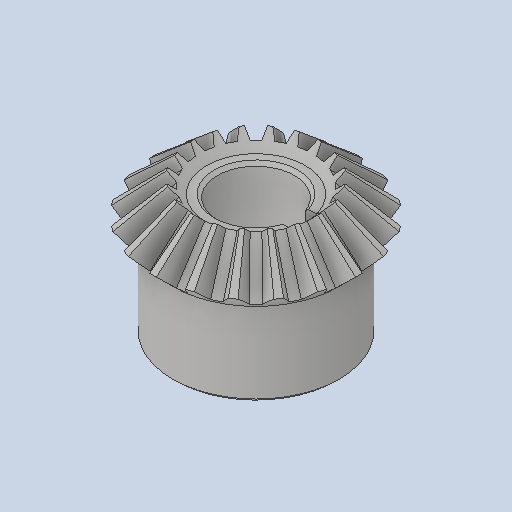
# Autodesk Inventor part: SMB1_5-201p_On
Saved by Autodesk Inventor 2025.2 (Build 292293000, 293)
## iProperties
Category: PARTsolutions
Company: KHK
Created: 2023-02-24
Part Number: SMB1_5-201p_On
Material: Generic
Catalog Web Link: www.cadenas.de
Description: SMB-
Vendor: KHK
Document SubType Name: Modeling
Designer: psAdmin
Manufacturer: KHK
Mass: 7.93706 g
Surface Area: 38.4961 cm^2
Volume: 7.93706 cm^3
Density: 1 g/cm^3
Appearance: PSOLRGB-175-175-175
PSOL_IDENT_0: {$CADENAS_DATA/23d-libs/khk/miter_gears/smb.prj},178 {VTYP=3D},{NB=SMB1.5-201p_On},{LINA=SMB1.5-20},
PSOL_IDENT_1: {NN=SMB},{DATE=06.10.2022 23:14:45},{GEOMDATE=24.04.2019 13:37:34},{VERSION=},{LINEID=300},{WBVAR=CO
PSOL_IDENT_2: MBINATION,TOOTH},{WBNUMERIC=}  {NB=SMB1.5-201p_On},{LINA=SMB1.5-20},{KT=DUMMY},{CN=SMB1.5-20},{COMBI
PSOL_IDENT_3: NATION=1},{VERS=2},{M=1.5},{Z=20},{A=12},{B=26},{C=30},{D=32.12},{E=30},{F=21.24},{G=16.06},{H=13.0}
PSOL_IDENT_4: ,{I=19},{J=8},{K=15.37},{L=49.80},{KYW=4x1.8},{KW=4},{KD=1.8},{TDM=6.50},{TS=M5},{S=B3},{PN=SMB1.5-2
PSOL_IDENT_5: 0},{WMF=B3004.WMF},{X=0.5},{Y=0.5},{TSNDM=5},{TOOTH=On}
NB: SMB1.5-201p_On
NN: SMB
NBSYN: $CN.$COMBINATION.p_$TOOTH.
LINA: SMB1.5-20
CATALOG: KHK
CN: SMB1.5-20
COMBINATION: Single
VERS: 2
M: 1.5
Z: 20
A: 12
B: 26
C: 30
D: 32.12
E: 30
F: 21.24
G: 16.06
H: 13
I: 19
J: 8
K: 15.37
L: 49.8
KYW: 4x1.8
KW: 4
KD: 1.8
TDM: 6.5
TS: M5
S: B3
PN: SMB1.5-20
WMF: B3004.WMF
X: 0.5
Y: 0.5
TSNDM: 5
TOOTH: On
SUPPLIER: KHK
ARTICLENO: SMB1.5-201p_On
BOMINFO: SMB1.5-20
CREATOR: CADENAS GmbH
Title: SMB1.5-20
Author: Cadenas PARTsolutions
Autodesk Inventor part; units mm, degrees
sketch "Sketch_6" plane through (0, -17, 0) normal (0, 1, 0) x (1, 0, 0)
  arc A0 (-0.5083, 20.2214) -> (-1.5864, 14.3695) centre (19.5954, 13.4924) ccw
  arc A1 (-1.5864, 14.3695) -> (-2.9317, 14.1564) centre (0, 0) ccw
  arc A2 (-2.9317, 14.1564) -> (-5.7653, 19.3888) centre (-22.8058, 6.7768) ccw
  arc A3 (-5.7653, 19.3888) -> (-6.7322, 19.0746) centre (0, 0) ccw
  arc A4 (-6.7322, 19.0746) -> (-5.9492, 13.176) centre (14.467, 18.8874) ccw
  arc A5 (-5.9492, 13.176) -> (-7.1627, 12.5576) centre (0, 0) ccw
  arc A6 (-7.1627, 12.5576) -> (-11.4746, 16.6582) centre (-23.7837, -0.6023) ccw
  arc A7 (-11.4746, 16.6582) -> (-12.2971, 16.0607) centre (0, 0) ccw
  arc A8 (-12.2971, 16.0607) -> (-9.7296, 10.6927) centre (7.9224, 22.4335) ccw
  arc A9 (-9.7296, 10.6927) -> (-10.6927, 9.7296) centre (0, 0) ccw
  arc A10 (-10.6927, 9.7296) -> (-16.0607, 12.2971) centre (-22.4335, -7.9224) ccw
  arc A11 (-16.0607, 12.2971) -> (-16.6582, 11.4746) centre (0, 0) ccw
  arc A12 (-16.6582, 11.4746) -> (-12.5576, 7.1627) centre (0.6023, 23.7837) ccw
  arc A13 (-12.5576, 7.1627) -> (-13.176, 5.9492) centre (0, 0) ccw
  arc A14 (-13.176, 5.9492) -> (-19.0746, 6.7322) centre (-18.8874, -14.467) ccw
  arc A15 (-19.0746, 6.7322) -> (-19.3888, 5.7653) centre (0, 0) ccw
  arc A16 (-19.3888, 5.7653) -> (-14.1564, 2.9317) centre (-6.7768, 22.8058) ccw
  arc A17 (-14.1564, 2.9317) -> (-14.3695, 1.5864) centre (0, 0) ccw
  arc A18 (-14.3695, 1.5864) -> (-20.2214, 0.5083) centre (-13.4924, -19.5954) ccw
  arc A19 (-20.2214, 0.5083) -> (-20.2214, -0.5083) centre (0, 0) ccw
  arc A20 (-20.2214, -0.5083) -> (-14.3695, -1.5864) centre (-13.4924, 19.5954) ccw
  arc A21 (-14.3695, -1.5864) -> (-14.1564, -2.9317) centre (0, 0) ccw
  arc A22 (-14.1564, -2.9317) -> (-19.3888, -5.7653) centre (-6.7768, -22.8058) ccw
  arc A23 (-19.3888, -5.7653) -> (-19.0746, -6.7322) centre (0, 0) ccw
  arc A24 (-19.0746, -6.7322) -> (-13.176, -5.9492) centre (-18.8874, 14.467) ccw
  arc A25 (-13.176, -5.9492) -> (-12.5576, -7.1627) centre (0, 0) ccw
  arc A26 (-12.5576, -7.1627) -> (-16.6582, -11.4746) centre (0.6023, -23.7837) ccw
  arc A27 (-16.6582, -11.4746) -> (-16.0607, -12.2971) centre (0, 0) ccw
  arc A28 (-16.0607, -12.2971) -> (-10.6927, -9.7296) centre (-22.4335, 7.9224) ccw
  arc A29 (-10.6927, -9.7296) -> (-9.7296, -10.6927) centre (0, 0) ccw
  arc A30 (-9.7296, -10.6927) -> (-12.2971, -16.0607) centre (7.9224, -22.4335) ccw
  arc A31 (-12.2971, -16.0607) -> (-11.4746, -16.6582) centre (0, 0) ccw
  arc A32 (-11.4746, -16.6582) -> (-7.1627, -12.5576) centre (-23.7837, 0.6023) ccw
  arc A33 (-7.1627, -12.5576) -> (-5.9492, -13.176) centre (0, 0) ccw
  arc A34 (-5.9492, -13.176) -> (-6.7322, -19.0746) centre (14.467, -18.8874) ccw
  arc A35 (-6.7322, -19.0746) -> (-5.7653, -19.3888) centre (0, 0) ccw
  arc A36 (-5.7653, -19.3888) -> (-2.9317, -14.1564) centre (-22.8058, -6.7768) ccw
  arc A37 (-2.9317, -14.1564) -> (-1.5864, -14.3695) centre (0, 0) ccw
  arc A38 (-1.5864, -14.3695) -> (-0.5083, -20.2214) centre (19.5954, -13.4924) ccw
  arc A39 (-0.5083, -20.2214) -> (0.5083, -20.2214) centre (0, 0) ccw
  arc A40 (0.5083, -20.2214) -> (1.5864, -14.3695) centre (-19.5954, -13.4924) ccw
  arc A41 (1.5864, -14.3695) -> (2.9317, -14.1564) centre (0, 0) ccw
  arc A42 (2.9317, -14.1564) -> (5.7653, -19.3888) centre (22.8058, -6.7768) ccw
  arc A43 (5.7653, -19.3888) -> (6.7322, -19.0746) centre (0, 0) ccw
  arc A44 (6.7322, -19.0746) -> (5.9492, -13.176) centre (-14.467, -18.8874) ccw
  arc A45 (5.9492, -13.176) -> (7.1627, -12.5576) centre (0, 0) ccw
  arc A46 (7.1627, -12.5576) -> (11.4746, -16.6582) centre (23.7837, 0.6023) ccw
  arc A47 (11.4746, -16.6582) -> (12.2971, -16.0607) centre (0, 0) ccw
  arc A48 (12.2971, -16.0607) -> (9.7296, -10.6927) centre (-7.9224, -22.4335) ccw
  arc A49 (9.7296, -10.6927) -> (10.6927, -9.7296) centre (0, 0) ccw
  arc A50 (10.6927, -9.7296) -> (16.0607, -12.2971) centre (22.4335, 7.9224) ccw
  arc A51 (16.0607, -12.2971) -> (16.6582, -11.4746) centre (0, 0) ccw
  arc A52 (16.6582, -11.4746) -> (12.5576, -7.1627) centre (-0.6023, -23.7837) ccw
  arc A53 (12.5576, -7.1627) -> (13.176, -5.9492) centre (0, 0) ccw
  arc A54 (13.176, -5.9492) -> (19.0746, -6.7322) centre (18.8874, 14.467) ccw
  arc A55 (19.0746, -6.7322) -> (19.3888, -5.7653) centre (0, 0) ccw
  arc A56 (19.3888, -5.7653) -> (14.1564, -2.9317) centre (6.7768, -22.8058) ccw
  arc A57 (14.1564, -2.9317) -> (14.3695, -1.5864) centre (0, 0) ccw
  arc A58 (14.3695, -1.5864) -> (20.2214, -0.5083) centre (13.4924, 19.5954) ccw
  arc A59 (20.2214, -0.5083) -> (20.2214, 0.5083) centre (0, 0) ccw
  arc A60 (20.2214, 0.5083) -> (14.3695, 1.5864) centre (13.4924, -19.5954) ccw
  arc A61 (14.3695, 1.5864) -> (14.1564, 2.9317) centre (0, 0) ccw
  arc A62 (14.1564, 2.9317) -> (19.3888, 5.7653) centre (6.7768, 22.8058) ccw
  arc A63 (19.3888, 5.7653) -> (19.0746, 6.7322) centre (0, 0) ccw
  arc A64 (19.0746, 6.7322) -> (13.176, 5.9492) centre (18.8874, -14.467) ccw
  arc A65 (13.176, 5.9492) -> (12.5576, 7.1627) centre (0, 0) ccw
  arc A66 (12.5576, 7.1627) -> (16.6582, 11.4746) centre (-0.6023, 23.7837) ccw
  arc A67 (16.6582, 11.4746) -> (16.0607, 12.2971) centre (0, 0) ccw
  arc A68 (16.0607, 12.2971) -> (10.6927, 9.7296) centre (22.4335, -7.9224) ccw
  arc A69 (10.6927, 9.7296) -> (9.7296, 10.6927) centre (0, 0) ccw
  arc A70 (9.7296, 10.6927) -> (12.2971, 16.0607) centre (-7.9224, 22.4335) ccw
  arc A71 (12.2971, 16.0607) -> (11.4746, 16.6582) centre (0, 0) ccw
  arc A72 (11.4746, 16.6582) -> (7.1627, 12.5576) centre (23.7837, -0.6023) ccw
  arc A73 (7.1627, 12.5576) -> (5.9492, 13.176) centre (0, 0) ccw
  arc A74 (5.9492, 13.176) -> (6.7322, 19.0746) centre (-14.467, 18.8874) ccw
  arc A75 (6.7322, 19.0746) -> (5.7653, 19.3888) centre (0, 0) ccw
  arc A76 (5.7653, 19.3888) -> (2.9317, 14.1564) centre (22.8058, 6.7768) ccw
  arc A77 (2.9317, 14.1564) -> (1.5864, 14.3695) centre (0, 0) ccw
  arc A78 (1.5864, 14.3695) -> (0.5083, 20.2214) centre (-19.5954, 13.4924) ccw
  arc A79 (0.5083, 20.2214) -> (-0.5083, 20.2214) centre (0, 0) ccw
  constraints: 160 point on circle, 80 centre point
sketch "Sketch_7" plane through (0, -8.76, 0) normal (0, 1, 0) x (1, 0, 0)
  arc A0 (-0.1963, 10.4116) -> (-0.6562, 5.9435) centre (20.5437, 6.0191) ccw
  arc A1 (-0.6562, 5.9435) -> (-1.2126, 5.8554) centre (0, 0) ccw
  arc A2 (-1.2126, 5.8554) -> (-3.0307, 9.9626) centre (-21.3982, -0.6238) ccw
  arc A3 (-3.0307, 9.9626) -> (-3.404, 9.8413) centre (0, 0) ccw
  arc A4 (-3.404, 9.8413) -> (-2.4607, 5.4499) centre (17.6782, 12.0729) ccw
  arc A5 (-2.4607, 5.4499) -> (-2.9627, 5.1941) centre (0, 0) ccw
  arc A6 (-2.9627, 5.1941) -> (-5.961, 8.5385) centre (-20.1582, -7.2057) ccw
  arc A7 (-5.961, 8.5385) -> (-6.2786, 8.3078) centre (0, 0) ccw
  arc A8 (-6.2786, 8.3078) -> (-4.0244, 4.4227) centre (13.0822, 16.9449) ccw
  arc A9 (-4.0244, 4.4227) -> (-4.4227, 4.0244) centre (0, 0) ccw
  arc A10 (-4.4227, 4.0244) -> (-8.3078, 6.2786) centre (-16.9449, -13.0822) ccw
  arc A11 (-8.3078, 6.2786) -> (-8.5385, 5.961) centre (0, 0) ccw
  arc A12 (-8.5385, 5.961) -> (-5.1941, 2.9627) centre (7.2057, 20.1582) ccw
  arc A13 (-5.1941, 2.9627) -> (-5.4499, 2.4607) centre (0, 0) ccw
  arc A14 (-5.4499, 2.4607) -> (-9.8413, 3.404) centre (-12.0729, -17.6782) ccw
  arc A15 (-9.8413, 3.404) -> (-9.9626, 3.0307) centre (0, 0) ccw
  arc A16 (-9.9626, 3.0307) -> (-5.8554, 1.2126) centre (0.6238, 21.3982) ccw
  arc A17 (-5.8554, 1.2126) -> (-5.9435, 0.6562) centre (0, 0) ccw
  arc A18 (-5.9435, 0.6562) -> (-10.4116, 0.1963) centre (-6.0191, -20.5437) ccw
  arc A19 (-10.4116, 0.1963) -> (-10.4116, -0.1963) centre (0, 0) ccw
  arc A20 (-10.4116, -0.1963) -> (-5.9435, -0.6562) centre (-6.0191, 20.5437) ccw
  arc A21 (-5.9435, -0.6562) -> (-5.8554, -1.2126) centre (0, 0) ccw
  arc A22 (-5.8554, -1.2126) -> (-9.9626, -3.0307) centre (0.6238, -21.3982) ccw
  arc A23 (-9.9626, -3.0307) -> (-9.8413, -3.404) centre (0, 0) ccw
  arc A24 (-9.8413, -3.404) -> (-5.4499, -2.4607) centre (-12.0729, 17.6782) ccw
  arc A25 (-5.4499, -2.4607) -> (-5.1941, -2.9627) centre (0, 0) ccw
  arc A26 (-5.1941, -2.9627) -> (-8.5385, -5.961) centre (7.2057, -20.1582) ccw
  arc A27 (-8.5385, -5.961) -> (-8.3078, -6.2786) centre (0, 0) ccw
  arc A28 (-8.3078, -6.2786) -> (-4.4227, -4.0244) centre (-16.9449, 13.0822) ccw
  arc A29 (-4.4227, -4.0244) -> (-4.0244, -4.4227) centre (0, 0) ccw
  arc A30 (-4.0244, -4.4227) -> (-6.2786, -8.3078) centre (13.0822, -16.9449) ccw
  arc A31 (-6.2786, -8.3078) -> (-5.961, -8.5385) centre (0, 0) ccw
  arc A32 (-5.961, -8.5385) -> (-2.9627, -5.1941) centre (-20.1582, 7.2057) ccw
  arc A33 (-2.9627, -5.1941) -> (-2.4607, -5.4499) centre (0, 0) ccw
  arc A34 (-2.4607, -5.4499) -> (-3.404, -9.8413) centre (17.6782, -12.0729) ccw
  arc A35 (-3.404, -9.8413) -> (-3.0307, -9.9626) centre (0, 0) ccw
  arc A36 (-3.0307, -9.9626) -> (-1.2126, -5.8554) centre (-21.3982, 0.6238) ccw
  arc A37 (-1.2126, -5.8554) -> (-0.6562, -5.9435) centre (0, 0) ccw
  arc A38 (-0.6562, -5.9435) -> (-0.1963, -10.4116) centre (20.5437, -6.0191) ccw
  arc A39 (-0.1963, -10.4116) -> (0.1963, -10.4116) centre (0, 0) ccw
  arc A40 (0.1963, -10.4116) -> (0.6562, -5.9435) centre (-20.5437, -6.0191) ccw
  arc A41 (0.6562, -5.9435) -> (1.2126, -5.8554) centre (0, 0) ccw
  arc A42 (1.2126, -5.8554) -> (3.0307, -9.9626) centre (21.3982, 0.6238) ccw
  arc A43 (3.0307, -9.9626) -> (3.404, -9.8413) centre (0, 0) ccw
  arc A44 (3.404, -9.8413) -> (2.4607, -5.4499) centre (-17.6782, -12.0729) ccw
  arc A45 (2.4607, -5.4499) -> (2.9627, -5.1941) centre (0, 0) ccw
  arc A46 (2.9627, -5.1941) -> (5.961, -8.5385) centre (20.1582, 7.2057) ccw
  arc A47 (5.961, -8.5385) -> (6.2786, -8.3078) centre (0, 0) ccw
  arc A48 (6.2786, -8.3078) -> (4.0244, -4.4227) centre (-13.0822, -16.9449) ccw
  arc A49 (4.0244, -4.4227) -> (4.4227, -4.0244) centre (0, 0) ccw
  arc A50 (4.4227, -4.0244) -> (8.3078, -6.2786) centre (16.9449, 13.0822) ccw
  arc A51 (8.3078, -6.2786) -> (8.5385, -5.961) centre (0, 0) ccw
  arc A52 (8.5385, -5.961) -> (5.1941, -2.9627) centre (-7.2057, -20.1582) ccw
  arc A53 (5.1941, -2.9627) -> (5.4499, -2.4607) centre (0, 0) ccw
  arc A54 (5.4499, -2.4607) -> (9.8413, -3.404) centre (12.0729, 17.6782) ccw
  arc A55 (9.8413, -3.404) -> (9.9626, -3.0307) centre (0, 0) ccw
  arc A56 (9.9626, -3.0307) -> (5.8554, -1.2126) centre (-0.6238, -21.3982) ccw
  arc A57 (5.8554, -1.2126) -> (5.9435, -0.6562) centre (0, 0) ccw
  arc A58 (5.9435, -0.6562) -> (10.4116, -0.1963) centre (6.0191, 20.5437) ccw
  arc A59 (10.4116, -0.1963) -> (10.4116, 0.1963) centre (0, 0) ccw
  arc A60 (10.4116, 0.1963) -> (5.9435, 0.6562) centre (6.0191, -20.5437) ccw
  arc A61 (5.9435, 0.6562) -> (5.8554, 1.2126) centre (0, 0) ccw
  arc A62 (5.8554, 1.2126) -> (9.9626, 3.0307) centre (-0.6238, 21.3982) ccw
  arc A63 (9.9626, 3.0307) -> (9.8413, 3.404) centre (0, 0) ccw
  arc A64 (9.8413, 3.404) -> (5.4499, 2.4607) centre (12.0729, -17.6782) ccw
  arc A65 (5.4499, 2.4607) -> (5.1941, 2.9627) centre (0, 0) ccw
  arc A66 (5.1941, 2.9627) -> (8.5385, 5.961) centre (-7.2057, 20.1582) ccw
  arc A67 (8.5385, 5.961) -> (8.3078, 6.2786) centre (0, 0) ccw
  arc A68 (8.3078, 6.2786) -> (4.4227, 4.0244) centre (16.9449, -13.0822) ccw
  arc A69 (4.4227, 4.0244) -> (4.0244, 4.4227) centre (0, 0) ccw
  arc A70 (4.0244, 4.4227) -> (6.2786, 8.3078) centre (-13.0822, 16.9449) ccw
  arc A71 (6.2786, 8.3078) -> (5.961, 8.5385) centre (0, 0) ccw
  arc A72 (5.961, 8.5385) -> (2.9627, 5.1941) centre (20.1582, -7.2057) ccw
  arc A73 (2.9627, 5.1941) -> (2.4607, 5.4499) centre (0, 0) ccw
  arc A74 (2.4607, 5.4499) -> (3.404, 9.8413) centre (-17.6782, 12.0729) ccw
  arc A75 (3.404, 9.8413) -> (3.0307, 9.9626) centre (0, 0) ccw
  arc A76 (3.0307, 9.9626) -> (1.2126, 5.8554) centre (21.3982, -0.6238) ccw
  arc A77 (1.2126, 5.8554) -> (0.6562, 5.9435) centre (0, 0) ccw
  arc A78 (0.6562, 5.9435) -> (0.1963, 10.4116) centre (-20.5437, 6.0191) ccw
  arc A79 (0.1963, 10.4116) -> (-0.1963, 10.4116) centre (0, 0) ccw
  constraints: 160 point on circle, 80 centre point
loft "Loft1" add profiles "Sketch_6", "Sketch_7"
sketch "Sketch_8" plane through (0, 0, 0) normal (0, 0, 1) x (1, 0, 0)
  line L0 (0, -30) -> (0, -8.76)
  line L1 (0, -11) -> (7.6863, -11)
  line L2 (7.6863, -11) -> (8.7582, -9.9281)
  line L3 (8.7582, -9.9281) -> (13.94, -16.06)
  line L4 (13.94, -16.06) -> (13, -17)
  line L5 (13, -17) -> (13, -29.5)
  line L6 (13, -29.5) -> (12.5, -30)
  line L7 (12.5, -30) -> (0, -30)
  line L8 (0, -30) -> (0, -11)
  constraints: 18 end point
revolve "Revolution1" add sketch "Sketch_8" angle 360 about axis through (0, -30, 0) along (0, -1, 0)
sketch "Sketch_9" plane through (0, 0, 0) normal (0, 0, 1) x (1, 0, 0)
  line L0 (0, -30) -> (0, 0)
  line L1 (0, 0) -> (32.12, 0)
  line L2 (32.12, 0) -> (32.12, -17)
  line L3 (32.12, -17) -> (13, -17)
  line L4 (13, -17) -> (16.06, -13.94)
  line L5 (16.06, -13.94) -> (9.9281, -8.7582)
  line L6 (9.9281, -8.7582) -> (7.6863, -11)
  line L7 (7.6863, -11) -> (6.5, -11)
  line L8 (6.5, -11) -> (6, -11.5)
  line L9 (6, -11.5) -> (6, -29.5)
  line L10 (6, -29.5) -> (6.5, -30)
  line L11 (6.5, -30) -> (0, -30)
  line L12 (0, -30) -> (0, 0)
  constraints: 26 end point
revolve "Revolution2" cut sketch "Sketch_9" angle 360 about axis through (0, -30, 0) along (0, -1, 0)
sketch "Sketch_4" plane through (0, -23.5, 0) normal (0, 1, 0) x (1, 0, 0)
  line L0 (0, 13) -> (0, 4.899)
  line L1 (0, 4.899) -> (-2.067, 4.899)
  line L2 (-2.067, 4.899) -> (-2.067, 12.567)
  line L3 (-2.067, 12.567) -> (-2.5, 13)
  line L4 (-2.5, 13) -> (0, 13)
  line L5 (0, 13) -> (0, 4.899)
  constraints: 12 end point
revolve "Revolution3" cut sketch "Sketch_4" angle 360 about axis through (0, -23.5, -13) along (0, 0, -1)
thread "Thread1" size "M5x0.8" class "6H" standard "ISO Metric profile" length 7.668
sketch "Sketch_5" plane through (0, -23.5, 0) normal (0, 1, 0) x (1, 0, 0)
  line L0 (0, -2) -> (7.8, -2)
  line L1 (7.8, -2) -> (7.8, 2)
  line L2 (7.8, 2) -> (0, 2)
  line L3 (0, 2) -> (0, -2)
  constraints: 8 end point
extrude "Extrusion1" cut sketch "Sketch_5" along normal mid plane 38
ref_plane "b_XY" through (0, 0, 0) normal (0, 0, 1) x (1, 0, 0)
ref_plane "b_YZ" through (0, 0, 0) normal (1, 0, 0) x (0, 1, 0)
ref_plane "b_ZX" through (0, 0, 0) normal (0, 1, 0) x (0, 0, 1)
ref_plane "bb_XY" through (0, 0, 0) normal (0, 1, 0) x (1, 0, 0)
ref_plane "bb_YZ" through (0, 0, 0) normal (1, 0, 0) x (0, 0, -1)
ref_plane "bb_ZX" through (0, 0, 0) normal (0, 0, -1) x (0, 1, 0)
body "Solid1"
